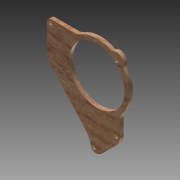
# Autodesk Inventor part: p1
Saved by Autodesk Inventor 2015 (Build 190159000, 159)
## iProperties
Created: 2016-02-03
Part Number: p1
Material: Generic
Document SubType Name: Modeling
Designer: david
Density: 1 g/cm^3
Appearance: Birch - Natural Polished
Mass: 12.4857 g
Surface Area: 88.0074 cm^2
Volume: 12.4857 cm^3
Author: david
Autodesk Inventor part; units mm, degrees
ref_plane "YZ Plane" through (0, 0, 0) normal (1, 0, 0) x (0, 1, 0)
ref_plane "XZ Plane" through (0, 0, 0) normal (0, 1, 0) x (-1, 0, 0)
ref_plane "XY Plane" through (0, 0, 0) normal (0, 0, 1) x (1, 0, 0)
sketch "Sketch1" plane through (0, 0, 0) normal (0, 1, 0) x (-1, 0, 0)
  line L0 (20, 45) -> (-20, 45)
  line L1 (-20, 45) -> (-20, -45)
  line L2 (-20, -45) -> (20, -45)
  line L3 (20, -45) -> (20, 45)
  line L4 (20, 45) -> (-20, -45) construction
  line L5 (-20, 45) -> (20, -45) construction
  line L6 (20, -45) -> (50, -45)
  line L7 (50, -45) -> (50, 45)
  line L8 (50, 45) -> (20, 45)
  line L9 (20, 45) -> (20, -45)
  point P0 (0, 0)
  dimension "d0" = 40
  dimension "d1" = 90
  dimension "d7" = 30
  dimension "d8" = 90
  constraints: 20 end point, 4 parallel, 2 horizontal, 2 midpoint, 2 perpendicular
  measures "d0" distance of L2.end L1.end
  measures "d1" distance of L1.end L0.end
  measures "d7" distance of L8.end L7.end
  measures "d8" distance of L7.end L6.end
extrude "Extrusion1" add sketch "Sketch1" along normal blind 3.6
sketch "Sketch3" plane through (0, 3.6, 0) normal (0, 1, 0) x (1, 0, 0)
  line L0 (-50, 45) -> (-50, -45) projected
  circle A0 centre (-30, 45) radius 22.5
  point P0 (0, 0)
  point P1 (20, 45)
  dimension "d37" = 20
  dimension "d38" = 45
  constraints: 1 centre point, 1 coincident
  measures "d37" distance from line of L0 point (-30, 45)
  measures "d38" diameter of A0
extrude "Extrusion3" cut sketch "Sketch3" against normal blind 10
fillet "Fillet2" radius 4 3 edges at (-50, 1.8, 45) (20, 1.8, 45) (-50, 1.8, -34.6922)
chamfer "Chamfer1" distance 20 angle 45 1 edges at (20, 1.8, -45)
fillet "Fillet4" radius 10 2 edges at (0, 1.8, -45) (20, 1.8, -25)
fillet "Fillet5" radius 5 1 edges at (-7.5, 1.8, -45)
sketch "Sketch9" plane through (0, 0, 0) normal (0, -1, 0) x (1, 0, 0)
  circle A0 centre (-46.5, 41.5) radius 1.5
  line L0 (-46, 45) -> (16, 45) projected
  line L1 (-50, -23.8754) -> (-50, 41) projected
  arc A1 (-50, -23.8754) -> (-43.5849, -27.064) centre (-46, -23.8754) ccw projected
  point P0 (0, 0)
  dimension "d70" = 3
  dimension "d72" = 3.5
  dimension "d73" = 3.5
  constraints: 1 centre point
  measures "d70" diameter of A0
  measures "d72" distance from line of L0 A0.centre
  measures "d73" distance from line of L1 A0.centre
extrude "Extrusion9" cut sketch "Sketch9" against normal blind 10
sketch "Sketch4" plane through (0, 3.6, 0) normal (0, 1, 0) x (1, 0, 0)
  circle A0 centre (-2, -20) radius 31
  line L0 (20, -41) -> (20, 45) projected
  line L1 (-46, -45) -> (16, -45) projected
  point P0 (0, 0)
  point P1 (20, 23.8754)
  dimension "d14" = 62
  dimension "d15" = 22
  dimension "d16" = 25
  constraints: 1 centre point
  measures "d14" diameter of A0
  measures "d15" distance from line of L0 A0.centre
  measures "d16" distance from line of L1 A0.centre
extrude "Extrusion4" add sketch "Sketch4" against normal blind 3.6
sketch "Sketch12" plane through (0, 3.6, 0) normal (0, 1, 0) x (1, 0, 0)
  arc A0 (19.8839, -41.9566) -> (20, 1.8403) centre (-2, -20) ccw projected
  circle A1 centre (-2, -20) radius 26.5
  point P0 (0, 0)
  dimension "d95" = 53
  constraints: 1 centre point, 1 coincident
  measures "d95" diameter of A1
extrude "Extrusion12" cut sketch "Sketch12" against normal blind 10
fillet "Fillet8" radius 10 2 edges at (-20.3303, 1.8, 45) (20, 1.8, -1.8403)
sketch "Sketch7" plane through (-32.64, 0, 1.0706) normal (0, -1, 0) x (1, 0, 0)
  circle A0 centre (27.64, -42.5706) radius 1.5
  circle A1 centre (49.14, -22.5706) radius 1.5
  circle A2 centre (49.14, 40.4294) radius 1.5
  line L0 (25.8579, -46.0706) -> (23.6643, -46.0706)
  line L1 (52.64, 41) -> (52.64, -20.8579)
  line L2 (-20, -45) -> (-20, 41)
  line L3 (-16, 43.9294) -> (46, 43.9294)
  line L4 (-13.36, 43.9294) -> (48.64, 43.9294) projected
  line L5 (52.64, 39.9294) -> (52.64, -21.9285) projected
  point P0 (0, 0)
  dimension "d56" = 3
  dimension "d53" = 3
  dimension "d50" = 3
  dimension "d58" = 3.5
  dimension "d55" = 3.5
  dimension "d57" = 25
  dimension "d54" = 20
  dimension "d52" = 3.5
  dimension "d51" = 3.5
  dimension "d62" = 0
  dimension "d63" = 0
  dimension "d79" = 90
  constraints: 8 end point, 3 centre point
  measures "d56" diameter of A0
  measures "d53" diameter of A1
  measures "d50" diameter of A2
  measures "d58" distance from line of L0 A0.centre
  measures "d55" distance from line of L1 A1.centre
  measures "d57" distance from line of L1 A0.centre
  measures "d54" vertical distance of A1.centre A0.centre
  measures "d52" distance from line of A2.centre L3
  measures "d51" distance from line of L1 A2.centre
  measures "d62" distance between parallel lines of L4 L3
  measures "d63" distance between parallel lines of L5 L1
  measures "d79" distance between parallel lines of L4 L0
extrude "Extrusion7" cut sketch "Sketch7" against normal blind 10
sketch "Sketch13" plane through (0, 0, 0) normal (0, -1, 0) x (1, 0, 0)
  circle A0 centre (16.5, 41.5) radius 1.5 projected
  arc A1 (19.9534, 34.8424) -> (9.4018, 43.9217) centre (16.5, 41.5) ccw
  circle A2 centre (-2, 20) radius 26.5 projected
  circle A3 centre (-2, 20) radius 26.5
  circle A4 centre (16.5, 41.5) radius 2.7131
  point P0 (0, 0)
  dimension "d97" = 15
  constraints: 4 point on circle, 3 centre point, 3 coincident
  measures "d97" diameter of A1
extrude "Extrusion13" add sketch "Sketch13" against normal blind 3.6 contours A2 A4 A1 | A2 A4 picked at (14.5458, 40.9715)
sketch "Sketch14" plane through (0, 0, 0) normal (0, -1, 0) x (1, 0, 0)
  arc A0 (-7.8959, -40.7978) -> (-43.5849, -27.064) centre (-30, -45) ccw projected
  line L0 (-13.2295, -30) -> (-50, 11.1246)
  line L1 (-50, -23.8754) -> (-50, 41) projected
  line L2 (-50, 11.1246) -> (-50, -45)
  line L3 (-50, -45) -> (-13.2295, -30)
  point P0 (0, 0)
  dimension "d100" = 35
  dimension "d101" = 15
  constraints: 6 end point, 1 point on circle, 1 point on line, 1 vertical
  measures "d100" distance of L0.end L1.start
  measures "d101" vertical distance of A0.centre L0.start
extrude "Extrusion14" cut sketch "Sketch14" against normal blind 3.6
fillet "Fillet9" radius 5 1 edges at (-50, 1.8, 11.1246)
body "Solid1"
